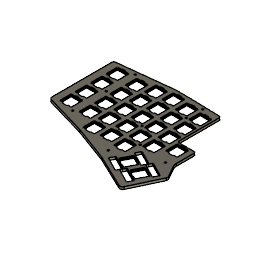
NestKeyboard (Autodesk Fusion 360 design; units mm, degrees)
part number: 2026-01-05-21-03-00-335
Autodesk Fusion 360 part; units mm, degrees
(part 1 of 4)
combine "Combine1" [no effect]
combine "Combine2" [no effect]
combine "Combine4" [no effect]
combine "Combine5" [no effect]
combine "Combine6" [no effect]
sketch "keyplate" plane through (0, 0, 0) normal (0, 0, 1) x (1, 0, 0)
  line L0 (65.8241, -96.8132) -> (65.8241, -83.8124)
  spline S0 degree 3 poles (65.8241, -83.8124) (65.8241, -83.5366) (65.6002, -83.3128) (65.3241, -83.3124) knots 0 0 0 0 1 1 1 1
  line L1 (65.3241, -83.3124) -> (52.3241, -83.3124)
  spline S1 degree 3 poles (52.3241, -83.3124) (52.0479, -83.3126) (51.8241, -83.5366) (51.824, -83.8124) knots 0 0 0 0 1 1 1 1
  line L2 (51.824, -83.8124) -> (51.824, -96.8132)
  spline S2 degree 3 poles (51.824, -96.8132) (51.8241, -97.0889) (52.0479, -97.3128) (52.3241, -97.3133) knots 0 0 0 0 1 1 1 1
  line L3 (52.3241, -97.3133) -> (65.3241, -97.3133)
  spline S3 degree 3 poles (65.3241, -97.3133) (65.6002, -97.3127) (65.8241, -97.0889) (65.8241, -96.8132) knots 0 0 0 0 1 1 1 1
  line L4 (84.8741, -94.432) -> (84.8741, -81.4312)
  spline S4 degree 3 poles (84.8741, -81.4312) (84.8741, -81.1554) (84.6502, -80.9315) (84.3741, -80.9311) knots 0 0 0 0 1 1 1 1
  line L5 (84.3741, -80.9311) -> (71.3741, -80.9311)
  spline S5 degree 3 poles (71.3741, -80.9311) (71.0979, -80.9314) (70.8741, -81.1554) (70.874, -81.4312) knots 0 0 0 0 1 1 1 1
  line L6 (70.874, -81.4312) -> (70.874, -94.432)
  spline S6 degree 3 poles (70.874, -94.432) (70.8741, -94.7077) (71.0979, -94.9315) (71.3741, -94.932) knots 0 0 0 0 1 1 1 1
  line L7 (71.3741, -94.932) -> (84.3741, -94.932)
  spline S7 degree 3 poles (84.3741, -94.932) (84.6502, -94.9315) (84.8741, -94.7077) (84.8741, -94.432) knots 0 0 0 0 1 1 1 1
  spline S8 degree 3 poles (103.4241, -97.3133) (103.7002, -97.3127) (103.9241, -97.0889) (103.9241, -96.8132) knots 0 0 0 0 1 1 1 1
  line L8 (103.9241, -96.8132) -> (103.9241, -83.8124)
  spline S9 degree 3 poles (103.9241, -83.8124) (103.9241, -83.5366) (103.7002, -83.3128) (103.4241, -83.3124) knots 0 0 0 0 1 1 1 1
  line L9 (103.4241, -83.3124) -> (90.4241, -83.3124)
  spline S10 degree 3 poles (90.4241, -83.3124) (90.1479, -83.3126) (89.9241, -83.5366) (89.924, -83.8124) knots 0 0 0 0 1 1 1 1
  line L10 (89.924, -83.8124) -> (89.924, -96.8132)
  spline S11 degree 3 poles (89.924, -96.8132) (89.9241, -97.0889) (90.1479, -97.3128) (90.4241, -97.3133) knots 0 0 0 0 1 1 1 1
  line L11 (90.4241, -97.3133) -> (103.4241, -97.3133)
  spline S12 degree 3 poles (114.051, -96.2404) (113.8049, -96.1145) (113.5038, -96.2123) (113.3784, -96.4581) knots 0 0 0 0 1 1 1 1
  line L12 (113.3784, -96.4581) -> (107.4766, -108.0414)
  spline S13 degree 3 poles (107.4766, -108.0414) (107.3512, -108.2875) (107.449, -108.5886) (107.6951, -108.7137) knots 0 0 0 0 1 1 1 1
  line L13 (107.6951, -108.7137) -> (119.2781, -114.616)
  spline S14 degree 3 poles (119.2781, -114.616) (119.5242, -114.7412) (119.8253, -114.6433) (119.9507, -114.397) knots 0 0 0 0 1 1 1 1
  line L14 (119.9507, -114.397) -> (125.8525, -102.8137)
  spline S15 degree 3 poles (125.8525, -102.8137) (125.9779, -102.5682) (125.8801, -102.2671) (125.634, -102.1414) knots 0 0 0 0 1 1 1 1
  line L15 (125.634, -102.1414) -> (114.051, -96.2404)
  line L16 (120.4218, -116.8097) -> (103.9464, -108.3923)
  spline S16 degree 3 poles (103.9464, -108.3923) (103.701, -108.2669) (103.3998, -108.3644) (103.2736, -108.61) knots 0 0 0 0 1 1 1 1
  line L17 (103.2736, -108.61) -> (100.5438, -113.9531)
  spline S17 degree 3 poles (100.5438, -113.9531) (100.4187, -114.1993) (100.5162, -114.5005) (100.7616, -114.6258) knots 0 0 0 0 1 1 1 1
  line L18 (100.7616, -114.6258) -> (117.2371, -123.0432)
  spline S18 degree 3 poles (117.2371, -123.0432) (117.4825, -123.1686) (117.7837, -123.0711) (117.9098, -122.8255) knots 0 0 0 0 1 1 1 1
  line L19 (117.9098, -122.8255) -> (120.6396, -117.4824)
  spline S19 degree 3 poles (120.6396, -117.4824) (120.7647, -117.2362) (120.6672, -116.935) (120.4218, -116.8097) knots 0 0 0 0 1 1 1 1
  line L20 (111.6094, -93.3658) -> (128.0874, -101.7782)
  spline S20 degree 3 poles (128.0874, -101.7782) (128.3328, -101.9035) (128.6339, -101.8059) (128.76, -101.5603) knots 0 0 0 0 1 1 1 1
  line L21 (128.76, -101.5603) -> (131.4882, -96.2164)
  spline S21 degree 3 poles (131.4882, -96.2164) (131.6132, -95.9702) (131.5156, -95.669) (131.2702, -95.5438) knots 0 0 0 0 1 1 1 1
  line L22 (131.2702, -95.5438) -> (114.7922, -87.1313)
  spline S22 degree 3 poles (114.7922, -87.1313) (114.5468, -87.006) (114.2456, -87.1036) (114.1196, -87.3492) knots 0 0 0 0 1 1 1 1
  line L23 (114.1196, -87.3492) -> (111.3913, -92.6932)
  spline S23 degree 3 poles (111.3913, -92.6932) (111.2663, -92.9394) (111.3639, -93.2405) (111.6094, -93.3658) knots 0 0 0 0 1 1 1 1
  line L24 (139.4813, -120.0656) -> (145.3833, -108.4837)
  spline S24 degree 3 poles (145.3833, -108.4837) (145.5086, -108.237) (145.4108, -107.9359) (145.1648, -107.8101) knots 0 0 0 0 1 1 1 1
  line L25 (145.1648, -107.8101) -> (133.5816, -101.909)
  spline S25 degree 3 poles (133.5816, -101.909) (133.3356, -101.7833) (133.0345, -101.8811) (132.9092, -102.1268) knots 0 0 0 0 1 1 1 1
  line L26 (132.9092, -102.1268) -> (127.0073, -113.71)
  spline S26 degree 3 poles (127.0073, -113.71) (126.8819, -113.9563) (126.9798, -114.2574) (127.2258, -114.3823) knots 0 0 0 0 1 1 1 1
  line L27 (127.2258, -114.3823) -> (138.8089, -120.2847)
  spline S27 degree 3 poles (138.8089, -120.2847) (139.0549, -120.41) (139.356, -120.3122) (139.4813, -120.0656) knots 0 0 0 0 1 1 1 1
  spline S28 degree 3 poles (130.9077, -98.3689) (130.7828, -98.6152) (130.8806, -98.9163) (131.1261, -99.0414) knots 0 0 0 0 1 1 1 1
  line L28 (131.1261, -99.0414) -> (147.6093, -107.4437)
  spline S29 degree 3 poles (147.6093, -107.4437) (147.8548, -107.5688) (148.1559, -107.4711) (148.2818, -107.2254) knots 0 0 0 0 1 1 1 1
  line L29 (148.2818, -107.2254) -> (151.0067, -101.8797)
  spline S30 degree 3 poles (151.0067, -101.8797) (151.1316, -101.6335) (151.0338, -101.3324) (150.7883, -101.2073) knots 0 0 0 0 1 1 1 1
  line L30 (150.7883, -101.2073) -> (134.3051, -92.805)
  spline S31 degree 3 poles (134.3051, -92.805) (134.0597, -92.6798) (133.7586, -92.7776) (133.6326, -93.0233) knots 0 0 0 0 1 1 1 1
  line L31 (133.6326, -93.0233) -> (130.9077, -98.3689)
  line L32 (120.2851, -120.3143) -> (136.7683, -128.7166)
  spline S32 degree 3 poles (136.7683, -128.7166) (137.0138, -128.8418) (137.3149, -128.744) (137.4408, -128.4982) knots 0 0 0 0 1 1 1 1
  line L33 (137.4408, -128.4982) -> (140.1657, -123.1527)
  spline S33 degree 3 poles (140.1657, -123.1527) (140.2906, -122.9064) (140.1928, -122.6053) (139.9473, -122.4801) knots 0 0 0 0 1 1 1 1
  line L34 (139.9473, -122.4801) -> (123.4642, -114.0778)
  spline S34 degree 3 poles (123.4642, -114.0778) (123.2186, -113.9527) (122.9175, -114.0505) (122.7916, -114.2962) knots 0 0 0 0 1 1 1 1
  line L35 (122.7916, -114.2962) -> (120.0667, -119.6418)
  spline S35 degree 3 poles (120.0667, -119.6418) (119.9418, -119.8881) (120.0396, -120.1892) (120.2851, -120.3143) knots 0 0 0 0 1 1 1 1
  spline S36 degree 3 poles (22.4616, -83.0258) (22.7377, -83.0252) (22.9616, -82.8014) (22.9616, -82.5257) knots 0 0 0 0 1 1 1 1
  line L36 (22.9616, -82.5257) -> (22.9616, -69.5249)
  spline S37 degree 3 poles (22.9616, -69.5249) (22.9616, -69.2491) (22.7377, -69.0253) (22.4616, -69.0249) knots 0 0 0 0 1 1 1 1
  line L37 (22.4616, -69.0249) -> (9.4616, -69.0249)
  spline S38 degree 3 poles (9.4616, -69.0249) (9.1854, -69.0254) (8.9616, -69.2491) (8.9616, -69.5249) knots 0 0 0 0 1 1 1 1
  line L38 (8.9616, -69.5249) -> (8.9616, -82.5257)
  spline S39 degree 3 poles (8.9616, -82.5257) (8.9616, -82.8014) (9.1854, -83.0253) (9.4616, -83.0258) knots 0 0 0 0 1 1 1 1
  line L39 (9.4616, -83.0258) -> (22.4616, -83.0258)
  line L40 (46.7741, -82.5257) -> (46.7741, -69.5249)
  spline S40 degree 3 poles (46.7741, -69.5249) (46.7741, -69.2491) (46.5502, -69.0253) (46.2741, -69.0249) knots 0 0 0 0 1 1 1 1
  line L41 (46.2741, -69.0249) -> (33.2741, -69.0249)
  spline S41 degree 3 poles (33.2741, -69.0249) (32.9979, -69.0254) (32.7741, -69.2491) (32.774, -69.5249) knots 0 0 0 0 1 1 1 1
  line L42 (32.774, -69.5249) -> (32.774, -82.5257)
  spline S42 degree 3 poles (32.774, -82.5257) (32.7741, -82.8014) (32.9979, -83.0253) (33.2741, -83.0258) knots 0 0 0 0 1 1 1 1
  line L43 (33.2741, -83.0258) -> (46.2741, -83.0258)
  spline S43 degree 3 poles (46.2741, -83.0258) (46.5502, -83.0252) (46.7741, -82.8014) (46.7741, -82.5257) knots 0 0 0 0 1 1 1 1
  line L44 (65.8241, -77.7632) -> (65.8241, -64.7624)
  spline S44 degree 3 poles (65.8241, -64.7624) (65.8241, -64.4866) (65.6002, -64.2628) (65.3241, -64.2624) knots 0 0 0 0 1 1 1 1
  line L45 (65.3241, -64.2624) -> (52.3241, -64.2624)
  spline S45 degree 3 poles (52.3241, -64.2624) (52.0479, -64.2629) (51.8241, -64.4866) (51.824, -64.7624) knots 0 0 0 0 1 1 1 1
  line L46 (51.824, -64.7624) -> (51.824, -77.7632)
  spline S46 degree 3 poles (51.824, -77.7632) (51.8241, -78.0389) (52.0479, -78.2628) (52.3241, -78.2633) knots 0 0 0 0 1 1 1 1
  line L47 (52.3241, -78.2633) -> (65.3241, -78.2633)
  spline S47 degree 3 poles (65.3241, -78.2633) (65.6002, -78.2627) (65.8241, -78.0389) (65.8241, -77.7632) knots 0 0 0 0 1 1 1 1
  line L48 (84.8741, -75.382) -> (84.8741, -62.3812)
  spline S48 degree 3 poles (84.8741, -62.3812) (84.8741, -62.1054) (84.6502, -61.8815) (84.3741, -61.8811) knots 0 0 0 0 1 1 1 1
  line L49 (84.3741, -61.8811) -> (71.3741, -61.8811)
  spline S49 degree 3 poles (71.3741, -61.8811) (71.0979, -61.8815) (70.8741, -62.1054) (70.874, -62.3812) knots 0 0 0 0 1 1 1 1
  line L50 (70.874, -62.3812) -> (70.874, -75.382)
  spline S50 degree 3 poles (70.874, -75.382) (70.8741, -75.6577) (71.0979, -75.8815) (71.3741, -75.882) knots 0 0 0 0 1 1 1 1
  line L51 (71.3741, -75.882) -> (84.3741, -75.882)
  spline S51 degree 3 poles (84.3741, -75.882) (84.6502, -75.8815) (84.8741, -75.6577) (84.8741, -75.382) knots 0 0 0 0 1 1 1 1
  line L52 (103.9241, -77.7632) -> (103.9241, -64.7624)
  spline S52 degree 3 poles (103.9241, -64.7624) (103.9241, -64.4866) (103.7002, -64.2628) (103.4241, -64.2624) knots 0 0 0 0 1 1 1 1
  line L53 (103.4241, -64.2624) -> (90.4241, -64.2624)
  spline S53 degree 3 poles (90.4241, -64.2624) (90.1479, -64.2629) (89.9241, -64.4866) (89.924, -64.7624) knots 0 0 0 0 1 1 1 1
  line L54 (89.924, -64.7624) -> (89.924, -77.7632)
  spline S54 degree 3 poles (89.924, -77.7632) (89.9241, -78.0389) (90.1479, -78.2628) (90.4241, -78.2633) knots 0 0 0 0 1 1 1 1
  line L55 (90.4241, -78.2633) -> (103.4241, -78.2633)
  spline S55 degree 3 poles (103.4241, -78.2633) (103.7002, -78.2627) (103.9241, -78.0389) (103.9241, -77.7632) knots 0 0 0 0 1 1 1 1
  spline S56 degree 3 poles (122.4741, -80.6445) (122.7502, -80.644) (122.9741, -80.4202) (122.9741, -80.1445) knots 0 0 0 0 1 1 1 1
  line L56 (122.9741, -80.1445) -> (122.9741, -67.1437)
  spline S57 degree 3 poles (122.9741, -67.1437) (122.9741, -66.8679) (122.7502, -66.644) (122.4741, -66.6436) knots 0 0 0 0 1 1 1 1
  line L57 (122.4741, -66.6436) -> (109.4741, -66.6436)
  spline S58 degree 3 poles (109.4741, -66.6436) (109.1979, -66.6442) (108.9741, -66.8679) (108.974, -67.1437) knots 0 0 0 0 1 1 1 1
  line L58 (108.974, -67.1437) -> (108.974, -80.1445)
  spline S59 degree 3 poles (108.974, -80.1445) (108.9741, -80.4202) (109.1979, -80.644) (109.4741, -80.6445) knots 0 0 0 0 1 1 1 1
  line L59 (109.4741, -80.6445) -> (122.4741, -80.6445)
  line L60 (142.0241, -70.6195) -> (142.0241, -57.6187)
  spline S60 degree 3 poles (142.0241, -57.6187) (142.0241, -57.3429) (141.8002, -57.119) (141.5241, -57.1186) knots 0 0 0 0 1 1 1 1
  line L61 (141.5241, -57.1186) -> (128.5241, -57.1186)
  spline S61 degree 3 poles (128.5241, -57.1186) (128.2479, -57.119) (128.0241, -57.3429) (128.024, -57.6187) knots 0 0 0 0 1 1 1 1
  line L62 (128.024, -57.6187) -> (128.024, -70.6195)
  spline S62 degree 3 poles (128.024, -70.6195) (128.0241, -70.8952) (128.2479, -71.119) (128.5241, -71.1195) knots 0 0 0 0 1 1 1 1
  line L63 (128.5241, -71.1195) -> (141.5241, -71.1195)
  spline S63 degree 3 poles (141.5241, -71.1195) (141.8002, -71.119) (142.0241, -70.8952) (142.0241, -70.6195) knots 0 0 0 0 1 1 1 1
  spline S64 degree 3 poles (22.4616, -63.9757) (22.7377, -63.9752) (22.9616, -63.7514) (22.9616, -63.4757) knots 0 0 0 0 1 1 1 1
  line L64 (22.9616, -63.4757) -> (22.9616, -50.4749)
  spline S65 degree 3 poles (22.9616, -50.4749) (22.9616, -50.1991) (22.7377, -49.9753) (22.4616, -49.9749) knots 0 0 0 0 1 1 1 1
  line L65 (22.4616, -49.9749) -> (9.4616, -49.9749)
  spline S66 degree 3 poles (9.4616, -49.9749) (9.1854, -49.9753) (8.9616, -50.1991) (8.9616, -50.4749) knots 0 0 0 0 1 1 1 1
  line L66 (8.9616, -50.4749) -> (8.9616, -63.4757)
  spline S67 degree 3 poles (8.9616, -63.4757) (8.9616, -63.7514) (9.1854, -63.9753) (9.4616, -63.9757) knots 0 0 0 0 1 1 1 1
  line L67 (9.4616, -63.9757) -> (22.4616, -63.9757)
  spline S68 degree 3 poles (46.2741, -63.9757) (46.5502, -63.9752) (46.7741, -63.7514) (46.7741, -63.4757) knots 0 0 0 0 1 1 1 1
  line L68 (46.7741, -63.4757) -> (46.7741, -50.4749)
  spline S69 degree 3 poles (46.7741, -50.4749) (46.7741, -50.1991) (46.5502, -49.9753) (46.2741, -49.9749) knots 0 0 0 0 1 1 1 1
  line L69 (46.2741, -49.9749) -> (33.2741, -49.9749)
  spline S70 degree 3 poles (33.2741, -49.9749) (32.9979, -49.9753) (32.7741, -50.1991) (32.774, -50.4749) knots 0 0 0 0 1 1 1 1
  line L70 (32.774, -50.4749) -> (32.774, -63.4757)
  spline S71 degree 3 poles (32.774, -63.4757) (32.7741, -63.7514) (32.9979, -63.9753) (33.2741, -63.9757) knots 0 0 0 0 1 1 1 1
  line L71 (33.2741, -63.9757) -> (46.2741, -63.9757)
  line L72 (65.8241, -58.7132) -> (65.8241, -45.7124)
  spline S72 degree 3 poles (65.8241, -45.7124) (65.8241, -45.4366) (65.6002, -45.2128) (65.3241, -45.2124) knots 0 0 0 0 1 1 1 1
  line L73 (65.3241, -45.2124) -> (52.3241, -45.2124)
  spline S73 degree 3 poles (52.3241, -45.2124) (52.0479, -45.2128) (51.8241, -45.4366) (51.824, -45.7124) knots 0 0 0 0 1 1 1 1
  line L74 (51.824, -45.7124) -> (51.824, -58.7132)
  spline S74 degree 3 poles (51.824, -58.7132) (51.8241, -58.9889) (52.0479, -59.2128) (52.3241, -59.2133) knots 0 0 0 0 1 1 1 1
  line L75 (52.3241, -59.2133) -> (65.3241, -59.2133)
  spline S75 degree 3 poles (65.3241, -59.2133) (65.6002, -59.2128) (65.8241, -58.9889) (65.8241, -58.7132) knots 0 0 0 0 1 1 1 1
  line L76 (84.8741, -56.332) -> (84.8741, -43.3312)
  spline S76 degree 3 poles (84.8741, -43.3312) (84.8741, -43.0554) (84.6502, -42.8315) (84.3741, -42.8311) knots 0 0 0 0 1 1 1 1
  line L77 (84.3741, -42.8311) -> (71.3741, -42.8311)
  spline S77 degree 3 poles (71.3741, -42.8311) (71.0979, -42.8315) (70.8741, -43.0554) (70.874, -43.3312) knots 0 0 0 0 1 1 1 1
  line L78 (70.874, -43.3312) -> (70.874, -56.332)
  spline S78 degree 3 poles (70.874, -56.332) (70.8741, -56.6077) (71.0979, -56.8315) (71.3741, -56.832) knots 0 0 0 0 1 1 1 1
  line L79 (71.3741, -56.832) -> (84.3741, -56.832)
  spline S79 degree 3 poles (84.3741, -56.832) (84.6502, -56.8315) (84.8741, -56.6077) (84.8741, -56.332) knots 0 0 0 0 1 1 1 1
  line L80 (103.9241, -58.7132) -> (103.9241, -45.7124)
  spline S80 degree 3 poles (103.9241, -45.7124) (103.9241, -45.4366) (103.7002, -45.2128) (103.4241, -45.2124) knots 0 0 0 0 1 1 1 1
  line L81 (103.4241, -45.2124) -> (90.4241, -45.2124)
  spline S81 degree 3 poles (90.4241, -45.2124) (90.1479, -45.2128) (89.9241, -45.4366) (89.924, -45.7124) knots 0 0 0 0 1 1 1 1
  line L82 (89.924, -45.7124) -> (89.924, -58.7132)
  spline S82 degree 3 poles (89.924, -58.7132) (89.9241, -58.9889) (90.1479, -59.2128) (90.4241, -59.2133) knots 0 0 0 0 1 1 1 1
  line L83 (90.4241, -59.2133) -> (103.4241, -59.2133)
  spline S83 degree 3 poles (103.4241, -59.2133) (103.7002, -59.2128) (103.9241, -58.9889) (103.9241, -58.7132) knots 0 0 0 0 1 1 1 1
  spline S84 degree 3 poles (122.4741, -61.5945) (122.7502, -61.594) (122.9741, -61.3702) (122.9741, -61.0945) knots 0 0 0 0 1 1 1 1
  line L84 (122.9741, -61.0945) -> (122.9741, -48.0937)
  spline S85 degree 3 poles (122.9741, -48.0937) (122.9741, -47.8179) (122.7502, -47.594) (122.4741, -47.5936) knots 0 0 0 0 1 1 1 1
  line L85 (122.4741, -47.5936) -> (109.4741, -47.5936)
  spline S86 degree 3 poles (109.4741, -47.5936) (109.1979, -47.594) (108.9741, -47.8179) (108.974, -48.0937) knots 0 0 0 0 1 1 1 1
  line L86 (108.974, -48.0937) -> (108.974, -61.0945)
  spline S87 degree 3 poles (108.974, -61.0945) (108.9741, -61.3702) (109.1979, -61.594) (109.4741, -61.5945) knots 0 0 0 0 1 1 1 1
  line L87 (109.4741, -61.5945) -> (122.4741, -61.5945)
  spline S88 degree 3 poles (22.4616, -44.9258) (22.7377, -44.9253) (22.9616, -44.7014) (22.9616, -44.4257) knots 0 0 0 0 1 1 1 1
  line L88 (22.9616, -44.4257) -> (22.9616, -31.4249)
  spline S89 degree 3 poles (22.9616, -31.4249) (22.9616, -31.1491) (22.7377, -30.9253) (22.4616, -30.9249) knots 0 0 0 0 1 1 1 1
  line L89 (22.4616, -30.9249) -> (9.4616, -30.9249)
  spline S90 degree 3 poles (9.4616, -30.9249) (9.1854, -30.9253) (8.9616, -31.1491) (8.9616, -31.4249) knots 0 0 0 0 1 1 1 1
  line L90 (8.9616, -31.4249) -> (8.9616, -44.4257)
  spline S91 degree 3 poles (8.9616, -44.4257) (8.9616, -44.7014) (9.1854, -44.9253) (9.4616, -44.9258) knots 0 0 0 0 1 1 1 1
  line L91 (9.4616, -44.9258) -> (22.4616, -44.9258)
  line L92 (46.7741, -44.4257) -> (46.7741, -31.4249)
  spline S92 degree 3 poles (46.7741, -31.4249) (46.7741, -31.1491) (46.5502, -30.9253) (46.2741, -30.9249) knots 0 0 0 0 1 1 1 1
  line L93 (46.2741, -30.9249) -> (33.2741, -30.9249)
  spline S93 degree 3 poles (33.2741, -30.9249) (32.9979, -30.9253) (32.7741, -31.1491) (32.774, -31.4249) knots 0 0 0 0 1 1 1 1
  line L94 (32.774, -31.4249) -> (32.774, -44.4257)
  spline S94 degree 3 poles (32.774, -44.4257) (32.7741, -44.7014) (32.9979, -44.9253) (33.2741, -44.9258) knots 0 0 0 0 1 1 1 1
  line L95 (33.2741, -44.9258) -> (46.2741, -44.9258)
  spline S95 degree 3 poles (46.2741, -44.9258) (46.5502, -44.9253) (46.7741, -44.7014) (46.7741, -44.4257) knots 0 0 0 0 1 1 1 1
  line L96 (65.8241, -39.6632) -> (65.8241, -26.6624)
  spline S96 degree 3 poles (65.8241, -26.6624) (65.8241, -26.3866) (65.6002, -26.1628) (65.3241, -26.1624) knots 0 0 0 0 1 1 1 1
  line L97 (65.3241, -26.1624) -> (52.3241, -26.1624)
  spline S97 degree 3 poles (52.3241, -26.1624) (52.0479, -26.1628) (51.8241, -26.3866) (51.824, -26.6624) knots 0 0 0 0 1 1 1 1
  line L98 (51.824, -26.6624) -> (51.824, -39.6632)
  spline S98 degree 3 poles (51.824, -39.6632) (51.8241, -39.9389) (52.0479, -40.1628) (52.3241, -40.1633) knots 0 0 0 0 1 1 1 1
  line L99 (52.3241, -40.1633) -> (65.3241, -40.1633)
  spline S99 degree 3 poles (65.3241, -40.1633) (65.6002, -40.1628) (65.8241, -39.9389) (65.8241, -39.6632) knots 0 0 0 0 1 1 1 1
  line L100 (84.8741, -37.282) -> (84.8741, -24.2812)
  spline S100 degree 3 poles (84.8741, -24.2812) (84.8741, -24.0054) (84.6502, -23.7815) (84.3741, -23.7811) knots 0 0 0 0 1 1 1 1
  line L101 (84.3741, -23.7811) -> (71.3741, -23.7811)
  spline S101 degree 3 poles (71.3741, -23.7811) (71.0979, -23.7815) (70.8741, -24.0054) (70.874, -24.2812) knots 0 0 0 0 1 1 1 1
  line L102 (70.874, -24.2812) -> (70.874, -37.282)
  spline S102 degree 3 poles (70.874, -37.282) (70.8741, -37.5577) (71.0979, -37.7815) (71.3741, -37.782) knots 0 0 0 0 1 1 1 1
  line L103 (71.3741, -37.782) -> (84.3741, -37.782)
  spline S103 degree 3 poles (84.3741, -37.782) (84.6502, -37.7815) (84.8741, -37.5577) (84.8741, -37.282) knots 0 0 0 0 1 1 1 1
  spline S104 degree 3 poles (103.4241, -40.1633) (103.7002, -40.1628) (103.9241, -39.9389) (103.9241, -39.6632) knots 0 0 0 0 1 1 1 1
  line L104 (103.9241, -39.6632) -> (103.9241, -26.6624)
  spline S105 degree 3 poles (103.9241, -26.6624) (103.9241, -26.3866) (103.7002, -26.1628) (103.4241, -26.1624) knots 0 0 0 0 1 1 1 1
  line L105 (103.4241, -26.1624) -> (90.4241, -26.1624)
  spline S106 degree 3 poles (90.4241, -26.1624) (90.1479, -26.1628) (89.9241, -26.3866) (89.924, -26.6624) knots 0 0 0 0 1 1 1 1
  line L106 (89.924, -26.6624) -> (89.924, -39.6632)
  spline S107 degree 3 poles (89.924, -39.6632) (89.9241, -39.9389) (90.1479, -40.1628) (90.4241, -40.1633) knots 0 0 0 0 1 1 1 1
  line L107 (90.4241, -40.1633) -> (103.4241, -40.1633)
  spline S108 degree 3 poles (122.4741, -42.5445) (122.7502, -42.544) (122.9741, -42.3202) (122.9741, -42.0445) knots 0 0 0 0 1 1 1 1
  line L108 (122.9741, -42.0445) -> (122.9741, -29.0437)
  spline S109 degree 3 poles (122.9741, -29.0437) (122.9741, -28.7679) (122.7502, -28.544) (122.4741, -28.5436) knots 0 0 0 0 1 1 1 1
  line L109 (122.4741, -28.5436) -> (109.4741, -28.5436)
  spline S110 degree 3 poles (109.4741, -28.5436) (109.1979, -28.544) (108.9741, -28.7679) (108.974, -29.0437) knots 0 0 0 0 1 1 1 1
  line L110 (108.974, -29.0437) -> (108.974, -42.0445)
  spline S111 degree 3 poles (108.974, -42.0445) (108.9741, -42.3202) (109.1979, -42.544) (109.4741, -42.5445) knots 0 0 0 0 1 1 1 1
  line L111 (109.4741, -42.5445) -> (122.4741, -42.5445)
  spline S112 degree 3 poles (22.4616, -25.8758) (22.7377, -25.8753) (22.9616, -25.6514) (22.9616, -25.3757) knots 0 0 0 0 1 1 1 1
  line L112 (22.9616, -25.3757) -> (22.9616, -12.3749)
  spline S113 degree 3 poles (22.9616, -12.3749) (22.9616, -12.0991) (22.7377, -11.8753) (22.4616, -11.8749) knots 0 0 0 0 1 1 1 1
  line L113 (22.4616, -11.8749) -> (9.4616, -11.8749)
  spline S114 degree 3 poles (9.4616, -11.8749) (9.1854, -11.8753) (8.9616, -12.0991) (8.9616, -12.3749) knots 0 0 0 0 1 1 1 1
  line L114 (8.9616, -12.3749) -> (8.9616, -25.3757)
  spline S115 degree 3 poles (8.9616, -25.3757) (8.9616, -25.6514) (9.1854, -25.8753) (9.4616, -25.8758) knots 0 0 0 0 1 1 1 1
  line L115 (9.4616, -25.8758) -> (22.4616, -25.8758)
  line L116 (46.7741, -25.3757) -> (46.7741, -12.3749)
  spline S116 degree 3 poles (46.7741, -12.3749) (46.7741, -12.0991) (46.5502, -11.8753) (46.2741, -11.8749) knots 0 0 0 0 1 1 1 1
  line L117 (46.2741, -11.8749) -> (33.2741, -11.8749)
  spline S117 degree 3 poles (33.2741, -11.8749) (32.9979, -11.8753) (32.7741, -12.0991) (32.774, -12.3749) knots 0 0 0 0 1 1 1 1
  line L118 (32.774, -12.3749) -> (32.774, -25.3757)
  spline S118 degree 3 poles (32.774, -25.3757) (32.7741, -25.6514) (32.9979, -25.8753) (33.2741, -25.8758) knots 0 0 0 0 1 1 1 1
  line L119 (33.2741, -25.8758) -> (46.2741, -25.8758)
  spline S119 degree 3 poles (46.2741, -25.8758) (46.5502, -25.8753) (46.7741, -25.6514) (46.7741, -25.3757) knots 0 0 0 0 1 1 1 1
  line L120 (65.8241, -20.6132) -> (65.8241, -7.6124)
  spline S120 degree 3 poles (65.8241, -7.6124) (65.8241, -7.3366) (65.6002, -7.1128) (65.3241, -7.1124) knots 0 0 0 0 1 1 1 1
  line L121 (65.3241, -7.1124) -> (52.3241, -7.1124)
  spline S121 degree 3 poles (52.3241, -7.1124) (52.0479, -7.1126) (51.8241, -7.3366) (51.824, -7.6124) knots 0 0 0 0 1 1 1 1
  line L122 (51.824, -7.6124) -> (51.824, -20.6132)
  spline S122 degree 3 poles (51.824, -20.6132) (51.8241, -20.8889) (52.0479, -21.1128) (52.3241, -21.1133) knots 0 0 0 0 1 1 1 1
  line L123 (52.3241, -21.1133) -> (65.3241, -21.1133)
  spline S123 degree 3 poles (65.3241, -21.1133) (65.6002, -21.1128) (65.8241, -20.8889) (65.8241, -20.6132) knots 0 0 0 0 1 1 1 1
  line L124 (84.8741, -18.232) -> (84.8741, -5.2312)
  spline S124 degree 3 poles (84.8741, -5.2312) (84.8741, -4.9554) (84.6502, -4.7315) (84.3741, -4.7311) knots 0 0 0 0 1 1 1 1
  line L125 (84.3741, -4.7311) -> (71.3741, -4.7311)
  spline S125 degree 3 poles (71.3741, -4.7311) (71.0979, -4.7317) (70.8741, -4.9554) (70.874, -5.2312) knots 0 0 0 0 1 1 1 1
  line L126 (70.874, -5.2312) -> (70.874, -18.232)
  spline S126 degree 3 poles (70.874, -18.232) (70.8741, -18.5077) (71.0979, -18.7315) (71.3741, -18.732) knots 0 0 0 0 1 1 1 1
  line L127 (71.3741, -18.732) -> (84.3741, -18.732)
  spline S127 degree 3 poles (84.3741, -18.732) (84.6502, -18.7315) (84.8741, -18.5077) (84.8741, -18.232) knots 0 0 0 0 1 1 1 1
  line L128 (103.9241, -20.6132) -> (103.9241, -7.6124)
  spline S128 degree 3 poles (103.9241, -7.6124) (103.9241, -7.3366) (103.7002, -7.1128) (103.4241, -7.1124) knots 0 0 0 0 1 1 1 1
  line L129 (103.4241, -7.1124) -> (90.4241, -7.1124)
  spline S129 degree 3 poles (90.4241, -7.1124) (90.1479, -7.1126) (89.9241, -7.3366) (89.924, -7.6124) knots 0 0 0 0 1 1 1 1
  line L130 (89.924, -7.6124) -> (89.924, -20.6132)
  spline S130 degree 3 poles (89.924, -20.6132) (89.9241, -20.8889) (90.1479, -21.1128) (90.4241, -21.1133) knots 0 0 0 0 1 1 1 1
  line L131 (90.4241, -21.1133) -> (103.4241, -21.1133)
  spline S131 degree 3 poles (103.4241, -21.1133) (103.7002, -21.1128) (103.9241, -20.8889) (103.9241, -20.6132) knots 0 0 0 0 1 1 1 1
  spline S132 degree 3 poles (122.4741, -23.4945) (122.7502, -23.494) (122.9741, -23.2702) (122.9741, -22.9945) knots 0 0 0 0 1 1 1 1
  line L132 (122.9741, -22.9945) -> (122.9741, -9.9937)
  spline S133 degree 3 poles (122.9741, -9.9937) (122.9741, -9.7179) (122.7502, -9.494) (122.4741, -9.4936) knots 0 0 0 0 1 1 1 1
  line L133 (122.4741, -9.4936) -> (109.4741, -9.4936)
  spline S134 degree 3 poles (109.4741, -9.4936) (109.1979, -9.4942) (108.9741, -9.7179) (108.974, -9.9937) knots 0 0 0 0 1 1 1 1
  line L134 (108.974, -9.9937) -> (108.974, -22.9945)
  spline S135 degree 3 poles (108.974, -22.9945) (108.9741, -23.2702) (109.1979, -23.494) (109.4741, -23.4945) knots 0 0 0 0 1 1 1 1
  line L135 (109.4741, -23.4945) -> (122.4741, -23.4945)
  circle A0 centre (27.6475, -44.3518) radius 1.1
  circle A1 centre (27.6475, -8.65) radius 1.1
  circle A2 centre (27.6475, -85.95) radius 1.1
  circle A3 centre (105.8014, -23.5848) radius 1.1
  circle A4 centre (105.9519, -80.7291) radius 1.1
  circle A5 centre (86.9775, -59.4768) radius 1.1
  circle A6 centre (92.2811, -106.4253) radius 1.1
  circle A7 centre (106.737, -4.0898) radius 1.1
  circle A8 centre (140.6317, -84.1371) radius 1.1
  line L136 (2.1623, -87.3399) -> (52.5628, -102.0002)
  line L137 (52.5628, -102.0002) -> (95.2143, -117.7482)
  line L138 (95.2143, -117.7482) -> (136.241, -137.3269)
  arc A9 (140.9605, -135.6379) -> (136.241, -137.3269) centre (137.7622, -134.1393) cw
  line L139 (140.9605, -135.6379) -> (157.6279, -100.0664)
  arc A10 (157.511, -97.1567) -> (157.6279, -100.0664) centre (154.7637, -98.7243) cw
  line L140 (157.511, -97.1567) -> (149.6607, -83.3982)
  arc A11 (149.6607, -83.3982) -> (148.4091, -78.6926) centre (157.9309, -78.6794) cw
  line L141 (148.4091, -78.6926) -> (148.3776, -56.0764)
  arc A12 (146.8839, -54.5848) -> (148.3776, -56.0764) centre (146.8839, -56.0785) cw
  line L142 (146.8839, -54.5848) -> (127.7559, -54.5848)
  arc A13 (127.7559, -54.5848) -> (125.9975, -52.8264) centre (127.7559, -52.8264) cw
  line L143 (125.9975, -52.8264) -> (125.9975, -2.6464)
  arc A14 (124.5064, -1.1127) -> (125.9975, -2.6464) centre (124.4632, -2.6464) cw
  line L144 (124.5064, -1.1127) -> (86.8308, -0.05)
  line L145 (86.8308, -0.05) -> (68.7069, -0.05)
  line L146 (68.7069, -0.05) -> (2.0445, -7.564)
  arc A15 (0.05, -9.7987) -> (2.0445, -7.564) centre (2.296, -9.7959) cw
  line L147 (0.05, -9.7987) -> (0.1425, -84.6522)
  arc A16 (2.1623, -87.3399) -> (0.1424, -84.6522) centre (2.9451, -84.6487) cw
  point P0 (28.7475, -44.3518)
  point P1 (28.7475, -8.65)
  point P2 (28.7475, -85.95)
  point P3 (106.9014, -23.5848)
  point P4 (107.0519, -80.7291)
  point P5 (88.0775, -59.4768)
  point P6 (93.3811, -106.4253)
  point P7 (107.837, -4.0898)
  point P8 (141.7317, -84.1371)
extrude "Extrude16" add sketch "keyplate" along normal blind 1.5 makes body 1
move_body "Move27" bodies 1 to x (1, 0, 0) y (0, 1, 0) z (0, 0, 1) at (0, 0, 1.5)
sketch "support" plane through (0, 0, 0) normal (0, 0, 1) x (1, 0, 0)
  line L0 (61.3126, -97.8124) -> (61.3127, -97.3129)
  line L1 (61.3127, -97.3129) -> (65.3126, -97.3123)
  spline S0 degree 3 poles (65.3126, -97.3123) (65.5888, -97.3118) (65.8126, -97.088) (65.8127, -96.8123) knots 0 0 0 0 1 1 1 1
  line L2 (65.8127, -96.8123) -> (65.8127, -83.8115)
  spline S1 degree 3 poles (65.8127, -83.8115) (65.8126, -83.5357) (65.5888, -83.3118) (65.3126, -83.3114) knots 0 0 0 0 1 1 1 1
  line L3 (65.3126, -83.3114) -> (61.3127, -83.3112)
  line L4 (61.3127, -83.3112) -> (61.3126, -82.8115)
  spline S2 degree 3 poles (61.3126, -82.8115) (61.3126, -82.5358) (61.0888, -82.312) (60.8126, -82.3115) knots 0 0 0 0 1 1 1 1
  line L5 (60.8126, -82.3115) -> (56.8126, -82.3115)
  spline S3 degree 3 poles (56.8126, -82.3115) (56.5365, -82.312) (56.3126, -82.5358) (56.3126, -82.8115) knots 0 0 0 0 1 1 1 1
  line L6 (56.3126, -82.8115) -> (56.3126, -83.3112)
  line L7 (56.3126, -83.3112) -> (52.3126, -83.3114)
  spline S4 degree 3 poles (52.3126, -83.3114) (52.0365, -83.3117) (51.8126, -83.5357) (51.8126, -83.8115) knots 0 0 0 0 1 1 1 1
  line L8 (51.8126, -83.8115) -> (51.8126, -96.8123)
  spline S5 degree 3 poles (51.8126, -96.8123) (51.8126, -97.088) (52.0365, -97.3119) (52.3126, -97.3123) knots 0 0 0 0 1 1 1 1
  line L9 (52.3126, -97.3123) -> (56.3126, -97.3129)
  line L10 (56.3126, -97.3129) -> (56.3126, -97.8124)
  spline S6 degree 3 poles (56.3126, -97.8124) (56.3126, -98.088) (56.5365, -98.3119) (56.8126, -98.3124) knots 0 0 0 0 1 1 1 1
  line L11 (56.8126, -98.3124) -> (60.8126, -98.3124)
  spline S7 degree 3 poles (60.8126, -98.3124) (61.0888, -98.3119) (61.3126, -98.088) (61.3126, -97.8124) knots 0 0 0 0 1 1 1 1
  line L12 (80.3626, -95.4312) -> (80.3627, -94.9316)
  line L13 (80.3627, -94.9316) -> (84.3626, -94.9311)
  spline S8 degree 3 poles (84.3626, -94.9311) (84.6388, -94.9305) (84.8626, -94.7067) (84.8627, -94.431) knots 0 0 0 0 1 1 1 1
  line L14 (84.8627, -94.431) -> (84.8627, -81.4302)
  spline S9 degree 3 poles (84.8627, -81.4302) (84.8626, -81.1545) (84.6388, -80.9306) (84.3626, -80.9302) knots 0 0 0 0 1 1 1 1
  line L15 (84.3626, -80.9302) -> (80.3627, -80.9299)
  line L16 (80.3627, -80.9299) -> (80.3626, -80.4303)
  spline S10 degree 3 poles (80.3626, -80.4303) (80.3626, -80.1546) (80.1388, -79.9307) (79.8626, -79.9303) knots 0 0 0 0 1 1 1 1
  line L17 (79.8626, -79.9303) -> (75.8626, -79.9303)
  spline S11 degree 3 poles (75.8626, -79.9303) (75.5865, -79.9308) (75.3626, -80.1546) (75.3626, -80.4303) knots 0 0 0 0 1 1 1 1
  line L18 (75.3626, -80.4303) -> (75.3626, -80.9299)
  line L19 (75.3626, -80.9299) -> (71.3626, -80.9302)
  spline S12 degree 3 poles (71.3626, -80.9302) (71.0865, -80.9305) (70.8626, -81.1545) (70.8626, -81.4302) knots 0 0 0 0 1 1 1 1
  line L20 (70.8626, -81.4302) -> (70.8626, -94.431)
  spline S13 degree 3 poles (70.8626, -94.431) (70.8626, -94.7067) (71.0865, -94.9306) (71.3626, -94.9311) knots 0 0 0 0 1 1 1 1
  line L21 (71.3626, -94.9311) -> (75.3626, -94.9316)
  line L22 (75.3626, -94.9316) -> (75.3626, -95.4312)
  spline S14 degree 3 poles (75.3626, -95.4312) (75.3626, -95.7068) (75.5865, -95.9306) (75.8626, -95.9312) knots 0 0 0 0 1 1 1 1
  line L23 (75.8626, -95.9312) -> (79.8626, -95.9312)
  spline S15 degree 3 poles (79.8626, -95.9312) (80.1388, -95.9307) (80.3626, -95.7068) (80.3626, -95.4312) knots 0 0 0 0 1 1 1 1
  line L24 (99.4126, -97.8124) -> (99.4127, -97.3129)
  line L25 (99.4127, -97.3129) -> (103.4126, -97.3123)
  spline S16 degree 3 poles (103.4126, -97.3123) (103.6888, -97.3118) (103.9126, -97.088) (103.9127, -96.8123) knots 0 0 0 0 1 1 1 1
  line L26 (103.9127, -96.8123) -> (103.9127, -83.8115)
  spline S17 degree 3 poles (103.9127, -83.8115) (103.9126, -83.5357) (103.6888, -83.3118) (103.4126, -83.3114) knots 0 0 0 0 1 1 1 1
  line L27 (103.4126, -83.3114) -> (99.4127, -83.3112)
  line L28 (99.4127, -83.3112) -> (99.4126, -82.8115)
  spline S18 degree 3 poles (99.4126, -82.8115) (99.4126, -82.5358) (99.1888, -82.312) (98.9126, -82.3115) knots 0 0 0 0 1 1 1 1
  line L29 (98.9126, -82.3115) -> (94.9126, -82.3115)
  spline S19 degree 3 poles (94.9126, -82.3115) (94.6365, -82.312) (94.4126, -82.5358) (94.4126, -82.8115) knots 0 0 0 0 1 1 1 1
  line L30 (94.4126, -82.8115) -> (94.4126, -83.3112)
  line L31 (94.4126, -83.3112) -> (90.4126, -83.3114)
  spline S20 degree 3 poles (90.4126, -83.3114) (90.1365, -83.3117) (89.9126, -83.5357) (89.9126, -83.8115) knots 0 0 0 0 1 1 1 1
  line L32 (89.9126, -83.8115) -> (89.9126, -96.8123)
  spline S21 degree 3 poles (89.9126, -96.8123) (89.9126, -97.088) (90.1365, -97.3119) (90.4126, -97.3123) knots 0 0 0 0 1 1 1 1
  line L33 (90.4126, -97.3123) -> (94.4126, -97.3129)
  line L34 (94.4126, -97.3129) -> (94.4126, -97.8124)
  spline S22 degree 3 poles (94.4126, -97.8124) (94.4126, -98.088) (94.6365, -98.3119) (94.9126, -98.3124) knots 0 0 0 0 1 1 1 1
  line L35 (94.9126, -98.3124) -> (98.9126, -98.3124)
  spline S23 degree 3 poles (98.9126, -98.3124) (99.1888, -98.3119) (99.4126, -98.088) (99.4126, -97.8124) knots 0 0 0 0 1 1 1 1
  line L36 (111.27, -111.6416) -> (114.834, -113.4571)
  spline S24 degree 3 poles (114.834, -113.4571) (115.0801, -113.5825) (115.3812, -113.4847) (115.5066, -113.2381) knots 0 0 0 0 1 1 1 1
  line L37 (115.5066, -113.2381) -> (115.7336, -112.7929)
  line L38 (115.7336, -112.7929) -> (119.2975, -114.6086)
  spline S25 degree 3 poles (119.2975, -114.6086) (119.5436, -114.7345) (119.8447, -114.6367) (119.9701, -114.3908) knots 0 0 0 0 1 1 1 1
  line L39 (119.9701, -114.3908) -> (125.8719, -102.8075)
  spline S26 degree 3 poles (125.8719, -102.8075) (125.9973, -102.5615) (125.8994, -102.2604) (125.6534, -102.1353) knots 0 0 0 0 1 1 1 1
  line L40 (125.6534, -102.1353) -> (122.0894, -100.3178)
  line L41 (122.0894, -100.3178) -> (122.3164, -99.8735)
  spline S27 degree 3 poles (122.3164, -99.8735) (122.4417, -99.6275) (122.3439, -99.3264) (122.0979, -99.2012) knots 0 0 0 0 1 1 1 1
  line L42 (122.0979, -99.2012) -> (118.5339, -97.3857)
  spline S28 degree 3 poles (118.5339, -97.3857) (118.2878, -97.2597) (117.9867, -97.3576) (117.8614, -97.6034) knots 0 0 0 0 1 1 1 1
  line L43 (117.8614, -97.6034) -> (117.6344, -98.0503)
  line L44 (117.6344, -98.0503) -> (114.0704, -96.2329)
  spline S29 degree 3 poles (114.0704, -96.2329) (113.8243, -96.1078) (113.5232, -96.2056) (113.3978, -96.452) knots 0 0 0 0 1 1 1 1
  line L45 (113.3978, -96.452) -> (107.496, -108.0352)
  spline S30 degree 3 poles (107.496, -108.0352) (107.3706, -108.2808) (107.4684, -108.5819) (107.7144, -108.7075) knots 0 0 0 0 1 1 1 1
  line L46 (107.7144, -108.7075) -> (111.2786, -110.5228)
  line L47 (111.2786, -110.5228) -> (111.0515, -110.9693)
  spline S31 degree 3 poles (111.0515, -110.9693) (110.9261, -111.2147) (111.0239, -111.5158) (111.27, -111.6416) knots 0 0 0 0 1 1 1 1
  line L48 (120.4218, -116.8097) -> (103.9464, -108.3923)
  spline S32 degree 3 poles (103.9464, -108.3923) (103.701, -108.2669) (103.3998, -108.3644) (103.2736, -108.61) knots 0 0 0 0 1 1 1 1
  line L49 (103.2736, -108.61) -> (100.5438, -113.9531)
  spline S33 degree 3 poles (100.5438, -113.9531) (100.4187, -114.1993) (100.5162, -114.5004) (100.7616, -114.6258) knots 0 0 0 0 1 1 1 1
  line L50 (100.7616, -114.6258) -> (117.2371, -123.0432)
  spline S34 degree 3 poles (117.2371, -123.0432) (117.4825, -123.1686) (117.7837, -123.0711) (117.9098, -122.8255) knots 0 0 0 0 1 1 1 1
  line L51 (117.9098, -122.8255) -> (120.6396, -117.4824)
  spline S35 degree 3 poles (120.6396, -117.4824) (120.7647, -117.2362) (120.6672, -116.935) (120.4218, -116.8097) knots 0 0 0 0 1 1 1 1
  line L52 (111.6094, -93.3658) -> (128.0874, -101.7782)
  spline S36 degree 3 poles (128.0874, -101.7782) (128.3328, -101.9035) (128.6339, -101.8059) (128.76, -101.5603) knots 0 0 0 0 1 1 1 1
  line L53 (128.76, -101.5603) -> (131.4882, -96.2164)
  spline S37 degree 3 poles (131.4882, -96.2164) (131.6132, -95.9702) (131.5156, -95.669) (131.2702, -95.5438) knots 0 0 0 0 1 1 1 1
  line L54 (131.2702, -95.5438) -> (114.7922, -87.1313)
  spline S38 degree 3 poles (114.7922, -87.1313) (114.5468, -87.006) (114.2456, -87.1036) (114.1196, -87.3492) knots 0 0 0 0 1 1 1 1
  line L55 (114.1196, -87.3492) -> (111.3913, -92.6932)
  spline S39 degree 3 poles (111.3913, -92.6932) (111.2663, -92.9394) (111.3639, -93.2405) (111.6094, -93.3658) knots 0 0 0 0 1 1 1 1
  line L56 (127.2338, -114.3905) -> (130.7978, -116.206)
  line L57 (130.7978, -116.206) -> (130.5708, -116.651)
  spline S40 degree 3 poles (130.5708, -116.651) (130.4455, -116.8975) (130.5433, -117.1986) (130.7893, -117.3246) knots 0 0 0 0 1 1 1 1
  line L58 (130.7893, -117.3246) -> (134.3533, -119.14)
  spline S41 degree 3 poles (134.3533, -119.14) (134.5994, -119.2653) (134.9005, -119.1674) (135.0259, -118.921) knots 0 0 0 0 1 1 1 1
  line L59 (135.0259, -118.921) -> (135.2529, -118.4761)
  line L60 (135.2529, -118.4761) -> (138.8168, -120.2915)
  spline S42 degree 3 poles (138.8168, -120.2915) (139.0629, -120.4172) (139.364, -120.3194) (139.4894, -120.0738) knots 0 0 0 0 1 1 1 1
  line L61 (139.4894, -120.0738) -> (145.3912, -108.4905)
  spline S43 degree 3 poles (145.3912, -108.4905) (145.5166, -108.2442) (145.4188, -107.9431) (145.1727, -107.8182) knots 0 0 0 0 1 1 1 1
  line L62 (145.1727, -107.8182) -> (141.6087, -106.001)
  line L63 (141.6087, -106.001) -> (141.8357, -105.5564)
  spline S44 degree 3 poles (141.8357, -105.5564) (141.9611, -105.3102) (141.8633, -105.0092) (141.6172, -104.8841) knots 0 0 0 0 1 1 1 1
  line L64 (141.6172, -104.8841) -> (138.0532, -103.0673)
  spline S45 degree 3 poles (138.0532, -103.0673) (137.8071, -102.9425) (137.5061, -103.0403) (137.3807, -103.2863) knots 0 0 0 0 1 1 1 1
  line L65 (137.3807, -103.2863) -> (137.1536, -103.7309)
  line L66 (137.1536, -103.7309) -> (133.5897, -101.9158)
  spline S46 degree 3 poles (133.5897, -101.9158) (133.3436, -101.7905) (133.0425, -101.8883) (132.9171, -102.1349) knots 0 0 0 0 1 1 1 1
  line L67 (132.9171, -102.1349) -> (127.0153, -113.7168)
  spline S47 degree 3 poles (127.0153, -113.7168) (126.8899, -113.9635) (126.9878, -114.2646) (127.2338, -114.3905) knots 0 0 0 0 1 1 1 1
  spline S48 degree 3 poles (130.9077, -98.3689) (130.7828, -98.6152) (130.8806, -98.9163) (131.1261, -99.0414) knots 0 0 0 0 1 1 1 1
  line L68 (131.1261, -99.0414) -> (147.6093, -107.4437)
  spline S49 degree 3 poles (147.6093, -107.4437) (147.8548, -107.5688) (148.1559, -107.4711) (148.2818, -107.2254) knots 0 0 0 0 1 1 1 1
  line L69 (148.2818, -107.2254) -> (151.0067, -101.8797)
  spline S50 degree 3 poles (151.0067, -101.8797) (151.1316, -101.6335) (151.0338, -101.3324) (150.7883, -101.2073) knots 0 0 0 0 1 1 1 1
  line L70 (150.7883, -101.2073) -> (134.3051, -92.805)
  spline S51 degree 3 poles (134.3051, -92.805) (134.0597, -92.6798) (133.7586, -92.7776) (133.6326, -93.0233) knots 0 0 0 0 1 1 1 1
  line L71 (133.6326, -93.0233) -> (130.9077, -98.3689)
  line L72 (120.2851, -120.3143) -> (136.7683, -128.7166)
  spline S52 degree 3 poles (136.7683, -128.7166) (137.0138, -128.8418) (137.3149, -128.744) (137.4408, -128.4982) knots 0 0 0 0 1 1 1 1
  line L73 (137.4408, -128.4982) -> (140.1657, -123.1527)
  spline S53 degree 3 poles (140.1657, -123.1527) (140.2906, -122.9064) (140.1928, -122.6053) (139.9473, -122.4801) knots 0 0 0 0 1 1 1 1
  line L74 (139.9473, -122.4801) -> (123.4642, -114.0778)
  spline S54 degree 3 poles (123.4642, -114.0778) (123.2186, -113.9527) (122.9175, -114.0505) (122.7916, -114.2962) knots 0 0 0 0 1 1 1 1
  line L75 (122.7916, -114.2962) -> (120.0667, -119.6418)
  spline S55 degree 3 poles (120.0667, -119.6418) (119.9418, -119.8881) (120.0396, -120.1892) (120.2851, -120.3143) knots 0 0 0 0 1 1 1 1
  spline S56 degree 3 poles (17.9501, -84.0249) (18.2263, -84.0244) (18.4501, -83.8005) (18.4501, -83.5249) knots 0 0 0 0 1 1 1 1
  line L76 (18.4501, -83.5249) -> (18.4501, -83.0254)
  line L77 (18.4501, -83.0254) -> (22.4501, -83.0248)
  spline S57 degree 3 poles (22.4501, -83.0248) (22.7263, -83.0243) (22.9501, -82.8005) (22.9501, -82.5248) knots 0 0 0 0 1 1 1 1
  line L78 (22.9501, -82.5248) -> (22.9501, -69.524)
  spline S58 degree 3 poles (22.9501, -69.524) (22.9501, -69.2482) (22.7263, -69.0243) (22.4501, -69.0239) knots 0 0 0 0 1 1 1 1
  line L79 (22.4501, -69.0239) -> (18.4501, -69.0236)
  line L80 (18.4501, -69.0236) -> (18.4501, -68.524)
  spline S59 degree 3 poles (18.4501, -68.524) (18.4501, -68.2483) (18.2263, -68.0244) (17.9501, -68.0239) knots 0 0 0 0 1 1 1 1
  line L81 (17.9501, -68.0239) -> (13.9501, -68.0239)
  spline S60 degree 3 poles (13.9501, -68.0239) (13.674, -68.0245) (13.4501, -68.2483) (13.4501, -68.524) knots 0 0 0 0 1 1 1 1
  line L82 (13.4501, -68.524) -> (13.4501, -69.0236)
  line L83 (13.4501, -69.0236) -> (9.4501, -69.0239)
  spline S61 degree 3 poles (9.4501, -69.0239) (9.174, -69.0241) (8.9501, -69.2481) (8.9501, -69.5239) knots 0 0 0 0 1 1 1 1
  line L84 (8.9501, -69.5239) -> (8.9501, -82.5247)
  spline S62 degree 3 poles (8.9501, -82.5247) (8.9501, -82.8004) (9.174, -83.0243) (9.4501, -83.0247) knots 0 0 0 0 1 1 1 1
  line L85 (9.4501, -83.0247) -> (13.4501, -83.0253)
  line L86 (13.4501, -83.0253) -> (13.4501, -83.5248)
  spline S63 degree 3 poles (13.4501, -83.5248) (13.4501, -83.8005) (13.674, -84.0243) (13.9501, -84.0249) knots 0 0 0 0 1 1 1 1
  line L87 (13.9501, -84.0249) -> (17.9501, -84.0249)
  line L88 (42.2626, -83.5249) -> (42.2627, -83.0254)
  line L89 (42.2627, -83.0254) -> (46.2626, -83.0248)
  spline S64 degree 3 poles (46.2626, -83.0248) (46.5388, -83.0243) (46.7626, -82.8005) (46.7627, -82.5248) knots 0 0 0 0 1 1 1 1
  line L90 (46.7627, -82.5248) -> (46.7627, -69.524)
  spline S65 degree 3 poles (46.7627, -69.524) (46.7626, -69.2482) (46.5388, -69.0243) (46.2626, -69.0239) knots 0 0 0 0 1 1 1 1
  line L91 (46.2626, -69.0239) -> (42.2627, -69.0237)
  line L92 (42.2627, -69.0237) -> (42.2626, -68.524)
  spline S66 degree 3 poles (42.2626, -68.524) (42.2626, -68.2483) (42.0388, -68.0245) (41.7626, -68.024) knots 0 0 0 0 1 1 1 1
  line L93 (41.7626, -68.024) -> (37.7626, -68.024)
  spline S67 degree 3 poles (37.7626, -68.024) (37.4865, -68.0245) (37.2626, -68.2483) (37.2626, -68.524) knots 0 0 0 0 1 1 1 1
  line L94 (37.2626, -68.524) -> (37.2626, -69.0237)
  line L95 (37.2626, -69.0237) -> (33.2626, -69.0239)
  spline S68 degree 3 poles (33.2626, -69.0239) (32.9865, -69.0242) (32.7626, -69.2482) (32.7626, -69.524) knots 0 0 0 0 1 1 1 1
  line L96 (32.7626, -69.524) -> (32.7626, -82.5248)
  spline S69 degree 3 poles (32.7626, -82.5248) (32.7626, -82.8005) (32.9865, -83.0244) (33.2626, -83.0248) knots 0 0 0 0 1 1 1 1
  line L97 (33.2626, -83.0248) -> (37.2626, -83.0254)
  line L98 (37.2626, -83.0254) -> (37.2626, -83.5249)
  spline S70 degree 3 poles (37.2626, -83.5249) (37.2626, -83.8005) (37.4865, -84.0244) (37.7626, -84.0249) knots 0 0 0 0 1 1 1 1
  line L99 (37.7626, -84.0249) -> (41.7626, -84.0249)
  spline S71 degree 3 poles (41.7626, -84.0249) (42.0388, -84.0244) (42.2626, -83.8005) (42.2626, -83.5249) knots 0 0 0 0 1 1 1 1
  line L100 (61.3126, -78.7624) -> (61.3127, -78.2629)
  line L101 (61.3127, -78.2629) -> (65.3126, -78.2623)
  spline S72 degree 3 poles (65.3126, -78.2623) (65.5888, -78.2618) (65.8126, -78.038) (65.8127, -77.7623) knots 0 0 0 0 1 1 1 1
  line L102 (65.8127, -77.7623) -> (65.8127, -64.7615)
  spline S73 degree 3 poles (65.8127, -64.7615) (65.8126, -64.4857) (65.5888, -64.2618) (65.3126, -64.2615) knots 0 0 0 0 1 1 1 1
  line L103 (65.3126, -64.2615) -> (61.3127, -64.2609)
  line L104 (61.3127, -64.2609) -> (61.3126, -63.7613)
  spline S74 degree 3 poles (61.3126, -63.7613) (61.3126, -63.4856) (61.0888, -63.2617) (60.8126, -63.2613) knots 0 0 0 0 1 1 1 1
  line L105 (60.8126, -63.2613) -> (56.8126, -63.2613)
  spline S75 degree 3 poles (56.8126, -63.2613) (56.5365, -63.2618) (56.3126, -63.4856) (56.3126, -63.7613) knots 0 0 0 0 1 1 1 1
  line L106 (56.3126, -63.7613) -> (56.3126, -64.2609)
  line L107 (56.3126, -64.2609) -> (52.3126, -64.2615)
  spline S76 degree 3 poles (52.3126, -64.2615) (52.0365, -64.2617) (51.8126, -64.4857) (51.8126, -64.7615) knots 0 0 0 0 1 1 1 1
  line L108 (51.8126, -64.7615) -> (51.8126, -77.7623)
  spline S77 degree 3 poles (51.8126, -77.7623) (51.8126, -78.038) (52.0365, -78.2619) (52.3126, -78.2623) knots 0 0 0 0 1 1 1 1
  line L109 (52.3126, -78.2623) -> (56.3126, -78.2629)
  line L110 (56.3126, -78.2629) -> (56.3126, -78.7624)
  spline S78 degree 3 poles (56.3126, -78.7624) (56.3126, -79.038) (56.5365, -79.2619) (56.8126, -79.2624) knots 0 0 0 0 1 1 1 1
  line L111 (56.8126, -79.2624) -> (60.8126, -79.2624)
  spline S79 degree 3 poles (60.8126, -79.2624) (61.0888, -79.2619) (61.3126, -79.038) (61.3126, -78.7624) knots 0 0 0 0 1 1 1 1
  line L112 (80.3626, -76.3812) -> (80.3627, -75.8816)
  line L113 (80.3627, -75.8816) -> (84.3626, -75.8811)
  spline S80 degree 3 poles (84.3626, -75.8811) (84.6388, -75.8805) (84.8626, -75.6567) (84.8627, -75.381) knots 0 0 0 0 1 1 1 1
  line L114 (84.8627, -75.381) -> (84.8627, -62.3802)
  spline S81 degree 3 poles (84.8627, -62.3802) (84.8626, -62.1045) (84.6388, -61.8806) (84.3626, -61.8802) knots 0 0 0 0 1 1 1 1
  line L115 (84.3626, -61.8802) -> (80.3627, -61.8797)
  line L116 (80.3627, -61.8797) -> (80.3626, -61.38)
  spline S82 degree 3 poles (80.3626, -61.38) (80.3626, -61.1043) (80.1388, -60.8805) (79.8626, -60.88) knots 0 0 0 0 1 1 1 1
  line L117 (79.8626, -60.88) -> (75.8626, -60.88)
  spline S83 degree 3 poles (75.8626, -60.88) (75.5865, -60.8805) (75.3626, -61.1043) (75.3626, -61.38) knots 0 0 0 0 1 1 1 1
  line L118 (75.3626, -61.38) -> (75.3626, -61.8797)
  line L119 (75.3626, -61.8797) -> (71.3626, -61.8802)
  spline S84 degree 3 poles (71.3626, -61.8802) (71.0865, -61.8805) (70.8626, -62.1045) (70.8626, -62.3802) knots 0 0 0 0 1 1 1 1
  line L120 (70.8626, -62.3802) -> (70.8626, -75.381)
  spline S85 degree 3 poles (70.8626, -75.381) (70.8626, -75.6567) (71.0865, -75.8806) (71.3626, -75.8811) knots 0 0 0 0 1 1 1 1
  line L121 (71.3626, -75.8811) -> (75.3626, -75.8816)
  line L122 (75.3626, -75.8816) -> (75.3626, -76.3812)
  spline S86 degree 3 poles (75.3626, -76.3812) (75.3626, -76.6568) (75.5865, -76.8806) (75.8626, -76.8812) knots 0 0 0 0 1 1 1 1
  line L123 (75.8626, -76.8812) -> (79.8626, -76.8812)
  spline S87 degree 3 poles (79.8626, -76.8812) (80.1388, -76.8807) (80.3626, -76.6568) (80.3626, -76.3812) knots 0 0 0 0 1 1 1 1
  line L124 (99.4126, -78.7624) -> (99.4127, -78.2629)
  line L125 (99.4127, -78.2629) -> (103.4126, -78.2623)
  spline S88 degree 3 poles (103.4126, -78.2623) (103.6888, -78.2618) (103.9126, -78.038) (103.9127, -77.7623) knots 0 0 0 0 1 1 1 1
  line L126 (103.9127, -77.7623) -> (103.9127, -64.7615)
  spline S89 degree 3 poles (103.9127, -64.7615) (103.9126, -64.4857) (103.6888, -64.2618) (103.4126, -64.2615) knots 0 0 0 0 1 1 1 1
  line L127 (103.4126, -64.2615) -> (99.4127, -64.2609)
  line L128 (99.4127, -64.2609) -> (99.4126, -63.7613)
  spline S90 degree 3 poles (99.4126, -63.7613) (99.4126, -63.4856) (99.1888, -63.2617) (98.9126, -63.2613) knots 0 0 0 0 1 1 1 1
  line L129 (98.9126, -63.2613) -> (94.9126, -63.2613)
  spline S91 degree 3 poles (94.9126, -63.2613) (94.6365, -63.2618) (94.4126, -63.4856) (94.4126, -63.7613) knots 0 0 0 0 1 1 1 1
  line L130 (94.4126, -63.7613) -> (94.4126, -64.2609)
  line L131 (94.4126, -64.2609) -> (90.4126, -64.2615)
  spline S92 degree 3 poles (90.4126, -64.2615) (90.1365, -64.2617) (89.9126, -64.4857) (89.9126, -64.7615) knots 0 0 0 0 1 1 1 1
  line L132 (89.9126, -64.7615) -> (89.9126, -77.7623)
  spline S93 degree 3 poles (89.9126, -77.7623) (89.9126, -78.038) (90.1365, -78.2619) (90.4126, -78.2623) knots 0 0 0 0 1 1 1 1
  line L133 (90.4126, -78.2623) -> (94.4126, -78.2629)
  line L134 (94.4126, -78.2629) -> (94.4126, -78.7624)
  spline S94 degree 3 poles (94.4126, -78.7624) (94.4126, -79.038) (94.6365, -79.2619) (94.9126, -79.2624) knots 0 0 0 0 1 1 1 1
  line L135 (94.9126, -79.2624) -> (98.9126, -79.2624)
  spline S95 degree 3 poles (98.9126, -79.2624) (99.1888, -79.2619) (99.4126, -79.038) (99.4126, -78.7624) knots 0 0 0 0 1 1 1 1
  line L136 (118.4626, -81.1437) -> (118.4627, -80.6441)
  line L137 (118.4627, -80.6441) -> (122.4626, -80.6436)
  spline S96 degree 3 poles (122.4626, -80.6436) (122.7388, -80.643) (122.9626, -80.4192) (122.9627, -80.1435) knots 0 0 0 0 1 1 1 1
  line L138 (122.9627, -80.1435) -> (122.9627, -67.1427)
  spline S97 degree 3 poles (122.9627, -67.1427) (122.9626, -66.867) (122.7388, -66.6431) (122.4626, -66.6427) knots 0 0 0 0 1 1 1 1
  line L139 (122.4626, -66.6427) -> (118.4627, -66.6422)
  line L140 (118.4627, -66.6422) -> (118.4626, -66.1425)
  spline S98 degree 3 poles (118.4626, -66.1425) (118.4626, -65.8668) (118.2388, -65.643) (117.9626, -65.6425) knots 0 0 0 0 1 1 1 1
  line L141 (117.9626, -65.6425) -> (113.9626, -65.6425)
  spline S99 degree 3 poles (113.9626, -65.6425) (113.6865, -65.643) (113.4626, -65.8668) (113.4626, -66.1425) knots 0 0 0 0 1 1 1 1
  line L142 (113.4626, -66.1425) -> (113.4626, -66.6422)
  line L143 (113.4626, -66.6422) -> (109.4626, -66.6427)
  spline S100 degree 3 poles (109.4626, -66.6427) (109.1865, -66.643) (108.9626, -66.867) (108.9626, -67.1427) knots 0 0 0 0 1 1 1 1
  line L144 (108.9626, -67.1427) -> (108.9626, -80.1435)
  spline S101 degree 3 poles (108.9626, -80.1435) (108.9626, -80.4192) (109.1865, -80.6431) (109.4626, -80.6436) knots 0 0 0 0 1 1 1 1
  line L145 (109.4626, -80.6436) -> (113.4626, -80.6441)
  line L146 (113.4626, -80.6441) -> (113.4626, -81.1437)
  spline S102 degree 3 poles (113.4626, -81.1437) (113.4626, -81.4193) (113.6865, -81.6431) (113.9626, -81.6437) knots 0 0 0 0 1 1 1 1
  line L147 (113.9626, -81.6437) -> (117.9626, -81.6437)
  spline S103 degree 3 poles (117.9626, -81.6437) (118.2388, -81.6432) (118.4626, -81.4193) (118.4626, -81.1437) knots 0 0 0 0 1 1 1 1
  line L148 (137.5127, -71.6187) -> (137.5127, -71.1191)
  line L149 (137.5127, -71.1191) -> (141.5126, -71.1186)